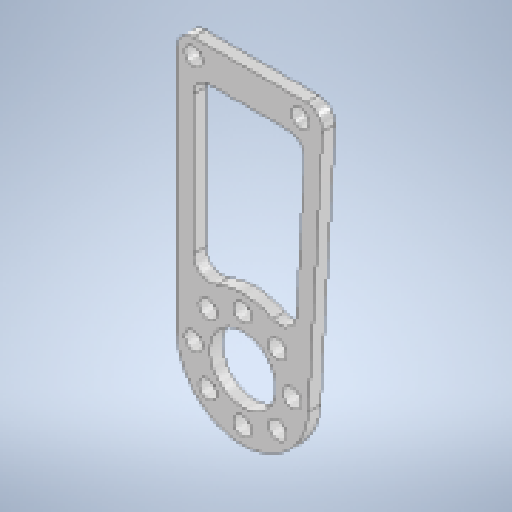
# Autodesk Inventor part: ude_new_new_1
Saved by Autodesk Inventor 2024 (Build 280153000, 153)
## iProperties
Created: 2024-01-03
Part Number: ude_new_new_1
Material: アルミニウム 2014-T4
Document SubType Name: Modeling
Designer: right
Density: 2.8 g/cm^3
Appearance: サテン
Mass: 1.20837 g
Surface Area: 9.7171 cm^2
Volume: 0.43156 cm^3
Author: right
Autodesk Inventor part; units mm, degrees
ref_plane "YZ Plane" through (0, 0, 0) normal (1, 0, 0) x (0, 1, 0)
ref_plane "XZ Plane" through (0, 0, 0) normal (0, 1, 0) x (-1, 0, 0)
ref_plane "XY Plane" through (0, 0, 0) normal (0, 0, 1) x (1, 0, 0)
sketch "スケッチ1" plane through (0, 0, 0) normal (0, 0, 1) x (1, 0, 0)
  line L0 (-9.2163, -10.1195) -> (-9.2163, -3.733) projected
  arc A0 (-9.2163, -10.1195) -> (-6.6163, -12.0274) centre (-7.2163, -10.1195) ccw projected
  arc A1 (5.1455, -12.36) -> (-6.6163, -12.0274) centre (-1.2163, -29.1983) ccw projected
  arc A2 (5.1455, -12.36) -> (7.8491, -10.6021) centre (5.8523, -10.4891) ccw projected
  line L1 (8.1822, -4.7177) -> (7.8491, -10.6021) projected
  line L2 (3.6894, -4.4634) -> (3.6601, -4.9812) projected
  arc A3 (1.4282, -6.8543) -> (3.6601, -4.9812) centre (1.6633, -4.8681) ccw projected
  arc A4 (1.4282, -6.8543) -> (-2.5938, -6.7405) centre (-1.2163, -29.1983) ccw projected
  arc A5 (-4.7163, -4.7443) -> (-2.5938, -6.7405) centre (-2.7163, -4.7443) ccw projected
  line L3 (-4.7163, -4.7443) -> (-4.7163, -3.9877) projected
  circle A6 centre (-1.2163, -29.1983) radius 4 projected
  arc A7 (5.7356, 31.6886) -> (3.7388, 33.8017) centre (3.7388, 31.8017) ccw projected
  line L4 (3.7388, 33.8017) -> (-2.7163, 33.8017) projected
  arc A8 (-2.7163, 33.8017) -> (-4.7163, 31.8017) centre (-2.7163, 31.8017) ccw projected
  line L5 (-4.7163, 31.8017) -> (-4.7163, -19.3115) projected
  line L6 (2.8369, -19.5251) -> (5.7356, 31.6886) projected
  circle A9 centre (7.7837, 36.3017) radius 1.1 projected
  circle A10 centre (-7.2163, 36.3017) radius 1.1 projected
  arc A11 (-5.4663, 59.6257) -> (-5.2163, 60.5939) centre (-7.2163, 60.5939) ccw projected
  arc A12 (-5.4663, 59.6257) -> (-5.7163, 58.6574) centre (-3.7163, 58.6574) ccw projected
  line L7 (-5.7163, 54.0245) -> (-5.7163, 58.6574) projected
  arc A13 (-5.7163, 54.0245) -> (-5.4663, 53.0563) centre (-3.7163, 54.0245) ccw projected
  arc A14 (-5.2163, 52.0881) -> (-5.4663, 53.0563) centre (-7.2163, 52.0881) ccw projected
  line L8 (-5.2163, 45.3017) -> (-5.2163, 52.0881) projected
  arc A15 (-5.2163, 45.3017) -> (-3.2163, 43.3017) centre (-3.2163, 45.3017) ccw projected
  line L9 (8.7837, 43.3017) -> (-3.2163, 43.3017) projected
  arc A16 (10.7805, 41.1886) -> (8.7837, 43.3017) centre (8.7837, 41.3017) ccw projected
  line L10 (6.771, -29.6504) -> (10.7805, 41.1886) projected
  arc A17 (-9.2163, -29.1983) -> (6.771, -29.6504) centre (-1.2163, -29.1983) ccw projected
  line L11 (-9.2163, 77.3017) -> (-9.2163, -29.1983) projected
  arc A18 (-5.2163, 77.3017) -> (-9.2163, 77.3017) centre (-7.2163, 77.3017) ccw projected
  line L12 (-5.2163, 76.0932) -> (-5.2163, 77.3017) projected
  arc A19 (-5.2163, 76.0932) -> (-5.2163, 65.5102) centre (0.7837, 70.8017) ccw projected
  line L13 (-5.2163, 60.5939) -> (-5.2163, 65.5102) projected
  circle A20 centre (-7.2163, 41.3017) radius 1.1 projected
  circle A21 centre (-7.2163, 77.3017) radius 1.1 projected
  circle A22 centre (8.7837, 41.3017) radius 1.1 projected
  circle A23 centre (-5.4589, -24.9557) radius 1.1 projected
  circle A24 centre (-1.2163, -23.1983) radius 1.1 projected
  circle A25 centre (3.0264, -24.9557) radius 1.1 projected
  circle A26 centre (4.7837, -29.1983) radius 1.1 projected
  circle A27 centre (3.0264, -33.441) radius 1.1 projected
  circle A28 centre (-1.2163, -35.1983) radius 1.1 projected
  circle A29 centre (-5.4589, -33.441) radius 1.1 projected
  circle A30 centre (-7.2163, -29.1983) radius 1.1 projected
  circle A31 centre (-1.2163, -29.1983) radius 4 projected
  line L14 (-9.2163, 2.8017) -> (8.6078, 2.8017)
  line L15 (-9.2163, -1.1983) -> (8.3814, -1.1983)
  line L16 (8.1822, -4.7177) -> (3.6894, -4.4634) projected
  line L17 (-4.7163, -3.9877) -> (-9.2163, -3.733) projected
  arc A32 (-4.7163, -19.3115) -> (-2.4163, -21.2888) centre (-2.7163, -19.3115) ccw projected
  arc A33 (0.4288, -21.3693) -> (-2.4163, -21.2888) centre (-1.2163, -29.1983) ccw projected
  arc A34 (0.4288, -21.3693) -> (2.8369, -19.5251) centre (0.8401, -19.412) ccw projected
  circle A35 centre (5.7837, 0.8017) radius 1.1 projected
  circle A36 centre (-7.2163, 0.8017) radius 1.1 projected
  point P0 (0, 0)
  point P1 (-9.2163, 11.5517)
  point P2 (-4.7163, 11.5517)
  point P3 (9.1031, 11.5517)
  point P4 (4.5959, 11.5517)
  point P5 (-9.2163, -4.5983)
  point P6 (8.1889, -4.5983)
  point P7 (-4.7163, -2.3057)
  point P8 (3.8115, -2.3057)
  point P9 (-3.4663, -6.5983)
  point P10 (2.6665, -6.5983)
  point P11 (8.0757, -6.5983)
  point P12 (-9.2163, -6.5983)
  point P13 (3.6817, -4.5983)
  point P14 (6.0725, -4.5983)
  point P15 (-4.7163, -4.5983)
  point P16 (-1.2163, -11.1983)
  point P17 (-8.9004, -11.1983)
  point P18 (7.7223, -11.1983)
  point P19 (3.2759, -11.7679)
  point P20 (-4.7163, -11.5419)
  point P21 (3.8742, -1.1983)
  point P22 (-4.7163, -4.7443)
  point P23 (-4.7163, -1.1983)
  dimension "d17" = 2
  dimension "d18" = 2
  constraints: 4 end point, 4 point on line, 1 parallel, 1 perpendicular
  measures "d17" distance from line of A36.centre L14
  measures "d18" distance from line of L15 A36.centre
extrude "押し出し1" add sketch "スケッチ1" along normal blind 1.5 contours L0 L17 L3 L5 A1 A0 | A0 A1 L5 A32 A33 A34 L6 A2 L10 A17 L11 | L11 L15 L5 L17 | L11 L14 L5 L15 | L5 L14 L6 L15 | L6 L2 L16 L1 A2 A1 | L15 L10 L16 L6 | L6 L14 L10 L15
sketch "スケッチ3" plane through (0, 0, 1.5) normal (0, 0, 1) x (1, 0, 0)
  arc A0 (-9.2163, -29.1983) -> (6.771, -29.6504) centre (-1.2163, -29.1983) ccw projected
  circle A1 centre (-1.2163, -35.1983) radius 1.1 projected
  circle A2 centre (-7.2163, -29.1983) radius 1.1 projected
  circle A3 centre (3.0264, -33.441) radius 1.1 projected
  circle A4 centre (4.7837, -29.1983) radius 1.1 projected
  circle A5 centre (-1.2163, -29.1983) radius 4 projected
  circle A6 centre (-5.4589, -33.441) radius 1.1 projected
  circle A7 centre (-1.2163, -23.1983) radius 1.1 projected
  circle A8 centre (-5.4589, -24.9557) radius 1.1 projected
  circle A9 centre (3.0264, -24.9557) radius 1.1 projected
  line L0 (-6.7163, 2.8017) -> (-6.7163, -29.1983)
  arc A10 (-6.7163, -29.1983) -> (4.275, -29.5091) centre (-1.2163, -29.1983) ccw
  line L1 (4.275, -29.5091) -> (6.1038, 2.8017)
  line L2 (6.1038, 2.8017) -> (-6.7163, 2.8017)
  line L3 (-6.7163, -1.1983) -> (5.8774, -1.1983)
  circle A11 centre (-1.2163, -29.1983) radius 8
  line L4 (6.771, -29.6504) -> (8.6078, 2.8017) projected
  line L5 (8.6078, 2.8017) -> (-9.2163, 2.8017) projected
  line L6 (-9.2163, 2.8017) -> (-9.2163, -29.1983) projected
  line L7 (-9.2163, 2.8017) -> (-9.2163, -29.1983) projected
  circle A12 centre (-7.2163, 0.8017) radius 1.1 projected
  point P0 (0, 0)
  point P1 (-6.7163, -23.3889)
  point P2 (4.6033, -23.7089)
  dimension "d12" = 16
  dimension "d19" = 2.5
  dimension "d21" = 2
  dimension "d23" = 2.5
  constraints: 8 end point, 3 point on line, 2 centre point, 2 horizontal, 2 point on circle, 1 coincident
  measures "d12" diameter of A11
  measures "d19" distance between parallel lines of L7 L0
  measures "d21" distance from line of L3 A12.centre
  measures "d23" distance between parallel lines of L4 L1
extrude "押し出し3" cut sketch "スケッチ3" against normal blind 1.5 contours L0 L3 L1 A11
fillet "フィレット4" radius 2 4 edges at (-6.7163, -23.3889, 0.75) (4.6033, -23.7089, 0.75) (5.8774, -1.1983, 0.75) (-6.7163, -1.1983, 0.75)
fillet "フィレット5" radius 2 2 edges at (-9.2163, 2.8017, 0.75) (8.6078, 2.8017, 0.75)
equation "\"d18\" = d17"
equation "\"d19\" = d23"
